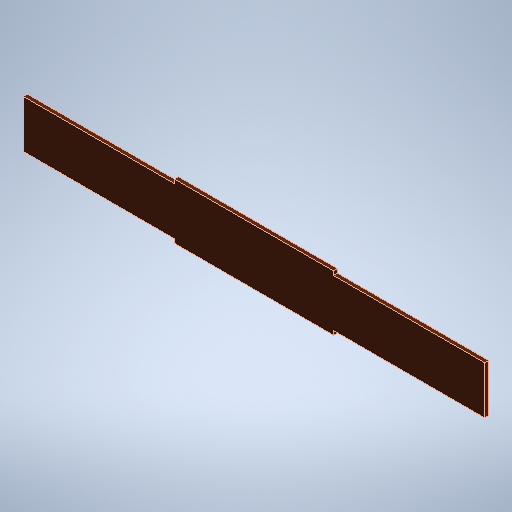
# Autodesk Inventor part: Table-Base Fixation
Saved by Autodesk Inventor 2025.4 (Build 294407000, 407)
## iProperties
Created: 2026-05-09
Part Number: Table-Base Fixation
Material: Generic
Document SubType Name: Sheet Metal
Designer: lenovo
Density: 1 g/cm^3
Sheet Metal Rule: Default_mm
Appearance: Default(1)
Author: lenovo
Autodesk Inventor part; units mm, degrees
ref_plane "YZ Plane" through (0, 0, 0) normal (1, 0, 0) x (0, 1, 0)
ref_plane "XZ Plane" through (0, 0, 0) normal (0, 1, 0) x (-1, 0, 0)
ref_plane "XY Plane" through (0, 0, 0) normal (0, 0, 1) x (1, 0, 0)
sketch "Sketch1" plane through (0, 0, 0) normal (0, 0, 1) x (1, 0, 0)
  line L0 (-290, -30) -> (290, -30)
  line L1 (290, -30) -> (290, 30)
  line L2 (290, 30) -> (-290, 30)
  line L3 (-290, 30) -> (-290, -30)
  line L4 (-290, -30) -> (290, 30) construction
  line L5 (290, -30) -> (-290, 30) construction
  line L6 (-100, 35) -> (100, 35)
  line L7 (100, 35) -> (100, 30)
  line L8 (100, 30) -> (-100, 30)
  line L9 (-100, 30) -> (-100, 35)
  line L10 (-100, 35) -> (100, 30) construction
  line L11 (100, 35) -> (-100, 30) construction
  line L12 (-290, 0) -> (290, 0)
  line L13 (-100, -35) -> (100, -35)
  line L14 (100, -35) -> (100, -30)
  line L15 (100, -30) -> (-100, -30)
  line L16 (-100, -30) -> (-100, -35)
  line L17 (-100, -35) -> (100, -30) construction
  line L18 (100, -35) -> (-100, -30) construction
  point P0 (0, 0)
  point P1 (0, 32.5)
  point P2 (0, 30)
  point P3 (0, -32.5)
  point P4 (0, -30)
  point P5 (-100, 30)
  point P6 (-100, -30)
  dimension "d0" = 580
  dimension "d1" = 60
  dimension "d2" = 5
  dimension "d3" = 200
  measures "d0" distance of L1.end L2.end
  measures "d1" distance of L0.end L1.end
  measures "d2" distance of L6.end L7.end
  measures "d3" distance of L6.start L6.end
extrude "Plate1" add sketch "Sketch1" along normal blind 5
equation "\"d4\" = Thickness"
equation "\"BendRadius\" = Thickness"
equation "\"BendReliefWidth\" = Thickness"
equation "\"BendReliefDepth\" = 0.5 * Thickness"
equation "\"TransitionRadius\" = BendRadius"
equation "\"JacobiRadiusSize\" = BendRadius"
equation "\"GapSize\" = Thickness"
equation "\"Thickness\" = 5"
body "Solid1"
